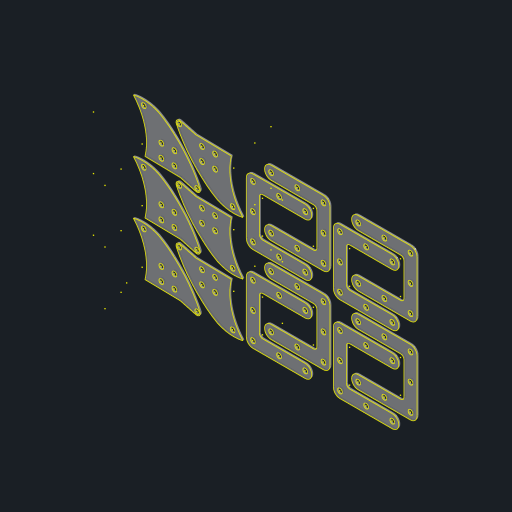
# Autodesk Inventor part: Nest.5-Sheet
Saved by Autodesk Inventor 2023 (Build 270158000, 158)
## iProperties
Created: 2023-05-16
Part Number: Nest.5-Sheet
Material: Polycarbonate, Clear
Document SubType Name: Modeling
Designer: reima
Density: 1.2 g/cm^3
Appearance: Polycarbonate - Clear
Author: reima
Autodesk Inventor part; units mm, degrees
ref_plane "YZ Plane" through (0, 0, 0) normal (1, 0, 0) x (0, 1, 0)
ref_plane "XZ Plane" through (0, 0, 0) normal (0, 1, 0) x (-1, 0, 0)
ref_plane "XY Plane" through (0, 0, 0) normal (0, 0, 1) x (1, 0, 0)
sketch "sleds sketch" plane through (0, 0, 0) normal (0, 0, 1) x (1, 0, 0)
  circle A0 centre (33.4038, 17.9574) radius 2.3114
  circle A1 centre (46.1038, 17.9574) radius 2.3114
  circle A2 centre (46.1038, 30.6574) radius 2.3114
  circle A3 centre (33.4038, 30.6574) radius 2.3114
  circle A4 centre (16.3571, 53.6521) radius 2.286
  circle A5 centre (68.0682, 9.9814) radius 2.159
  arc A6 (31.137, 55.194) -> (6.35, 57.7528) centre (15.0465, 20.661) ccw
  arc A7 (45.8139, 44.5419) -> (31.137, 55.194) centre (-5.4134, -10.6039) ccw
  arc A8 (70.9384, 11.3388) -> (45.8139, 44.5419) centre (-21.0694, -32.1754) ccw
  arc A9 (67.2386, 6.9167) -> (70.9384, 11.3388) centre (68.0682, 9.9814) ccw
  line L0 (67.2386, 6.9167) -> (51.9362, 11.059)
  line L1 (51.9362, 11.059) -> (17.5779, 11.7169)
  arc A10 (17.5779, 11.7169) -> (6.35, 57.7528) centre (-32.185, 23.9671) ccw
  constraints: 11 centre point, 10 point on circle, 4 end point
extrude "sleds extrude" add sketch "sleds sketch" along normal blind 1.5875
sketch "sleds (#2) sketch" plane through (0, 0, 0) normal (0, 0, 1) x (1, 0, 0)
  circle A0 centre (33.4038, 69.7529) radius 2.3114
  circle A1 centre (46.1038, 69.7529) radius 2.3114
  circle A2 centre (46.1038, 82.4529) radius 2.3114
  circle A3 centre (33.4038, 82.4529) radius 2.3114
  circle A4 centre (16.3571, 105.4475) radius 2.286
  circle A5 centre (68.0682, 61.7769) radius 2.159
  arc A6 (31.137, 106.9895) -> (6.35, 109.5483) centre (15.0465, 72.4565) ccw
  arc A7 (45.8139, 96.3374) -> (31.137, 106.9895) centre (-5.4134, 41.1916) ccw
  arc A8 (70.9384, 63.1343) -> (45.8139, 96.3374) centre (-21.0694, 19.6201) ccw
  arc A9 (67.2386, 58.7122) -> (70.9384, 63.1343) centre (68.0682, 61.7769) ccw
  line L0 (67.2386, 58.7122) -> (51.9362, 62.8545)
  line L1 (51.9362, 62.8545) -> (17.5779, 63.5124)
  arc A10 (17.5779, 63.5124) -> (6.35, 109.5483) centre (-32.185, 75.7626) ccw
  constraints: 11 centre point, 10 point on circle, 4 end point
extrude "sleds (#2) extrude" add sketch "sleds (#2) sketch" along normal blind 1.5875 separate body
sketch "sleds (#3) sketch" plane through (0, 0, 0) normal (0, 0, 1) x (1, 0, 0)
  circle A0 centre (33.4038, 121.5484) radius 2.3114
  circle A1 centre (46.1038, 121.5484) radius 2.3114
  circle A2 centre (46.1038, 134.2484) radius 2.3114
  circle A3 centre (33.4038, 134.2484) radius 2.3114
  circle A4 centre (16.3571, 157.243) radius 2.286
  circle A5 centre (68.0682, 113.5724) radius 2.159
  arc A6 (31.137, 158.785) -> (6.35, 161.3438) centre (15.0465, 124.252) ccw
  arc A7 (45.8139, 148.1329) -> (31.137, 158.785) centre (-5.4134, 92.9871) ccw
  arc A8 (70.9384, 114.9298) -> (45.8139, 148.1329) centre (-21.0694, 71.4156) ccw
  arc A9 (67.2386, 110.5077) -> (70.9384, 114.9298) centre (68.0682, 113.5724) ccw
  line L0 (67.2386, 110.5077) -> (51.9362, 114.6499)
  line L1 (51.9362, 114.6499) -> (17.5779, 115.3079)
  arc A10 (17.5779, 115.3079) -> (6.35, 161.3438) centre (-32.185, 127.5581) ccw
  constraints: 11 centre point, 10 point on circle, 4 end point
extrude "sleds (#3) extrude" add sketch "sleds (#3) sketch" along normal blind 1.5875 separate body
sketch "sleds (#4) sketch" plane through (0, 0, 0) normal (0, 0, 1) x (1, 0, 0)
  circle A0 centre (85.5586, 47.6077) radius 2.3114
  circle A1 centre (72.8586, 47.6077) radius 2.3114
  circle A2 centre (72.8586, 34.9077) radius 2.3114
  circle A3 centre (85.5586, 34.9077) radius 2.3114
  circle A4 centre (102.6053, 11.913) radius 2.286
  circle A5 centre (50.8942, 55.5837) radius 2.159
  arc A6 (87.8254, 10.3711) -> (112.6124, 7.8123) centre (103.9159, 44.9041) ccw
  arc A7 (73.1485, 21.0232) -> (87.8254, 10.3711) centre (124.3758, 76.169) ccw
  arc A8 (48.024, 54.2263) -> (73.1485, 21.0232) centre (140.0318, 97.7405) ccw
  arc A9 (51.7238, 58.6484) -> (48.024, 54.2263) centre (50.8942, 55.5837) ccw
  line L0 (51.7238, 58.6484) -> (67.0262, 54.5061)
  line L1 (67.0262, 54.5061) -> (101.3845, 53.8482)
  arc A10 (101.3845, 53.8482) -> (112.6124, 7.8123) centre (151.1474, 41.598) ccw
  constraints: 11 centre point, 10 point on circle, 4 end point
extrude "sleds (#4) extrude" add sketch "sleds (#4) sketch" along normal blind 1.5875 separate body
sketch "sleds (#5) sketch" plane through (0, 0, 0) normal (0, 0, 1) x (1, 0, 0)
  circle A0 centre (85.5586, 99.4032) radius 2.3114
  circle A1 centre (72.8586, 99.4032) radius 2.3114
  circle A2 centre (72.8586, 86.7032) radius 2.3114
  circle A3 centre (85.5586, 86.7032) radius 2.3114
  circle A4 centre (102.6053, 63.7085) radius 2.286
  circle A5 centre (50.8942, 107.3792) radius 2.159
  arc A6 (87.8254, 62.1666) -> (112.6124, 59.6077) centre (103.9159, 96.6996) ccw
  arc A7 (73.1485, 72.8187) -> (87.8254, 62.1666) centre (124.3758, 127.9645) ccw
  arc A8 (48.024, 106.0218) -> (73.1485, 72.8187) centre (140.0318, 149.536) ccw
  arc A9 (51.7238, 110.4439) -> (48.024, 106.0218) centre (50.8942, 107.3792) ccw
  line L0 (51.7238, 110.4439) -> (67.0262, 106.3016)
  line L1 (67.0262, 106.3016) -> (101.3845, 105.6437)
  arc A10 (101.3845, 105.6437) -> (112.6124, 59.6077) centre (151.1474, 93.3934) ccw
  constraints: 11 centre point, 10 point on circle, 4 end point
extrude "sleds (#5) extrude" add sketch "sleds (#5) sketch" along normal blind 1.5875 separate body
sketch "sleds (#6) sketch" plane through (0, 0, 0) normal (0, 0, 1) x (1, 0, 0)
  circle A0 centre (85.5586, 151.1987) radius 2.3114
  circle A1 centre (72.8586, 151.1987) radius 2.3114
  circle A2 centre (72.8586, 138.4987) radius 2.3114
  circle A3 centre (85.5586, 138.4987) radius 2.3114
  circle A4 centre (102.6053, 115.504) radius 2.286
  circle A5 centre (50.8942, 159.1747) radius 2.159
  arc A6 (87.8254, 113.9621) -> (112.6124, 111.4032) centre (103.9159, 148.4951) ccw
  arc A7 (73.1485, 124.6142) -> (87.8254, 113.9621) centre (124.3758, 179.76) ccw
  arc A8 (48.024, 157.8173) -> (73.1485, 124.6142) centre (140.0318, 201.3315) ccw
  arc A9 (51.7238, 162.2394) -> (48.024, 157.8173) centre (50.8942, 159.1747) ccw
  line L0 (51.7238, 162.2394) -> (67.0262, 158.0971)
  line L1 (67.0262, 158.0971) -> (101.3845, 157.4392)
  arc A10 (101.3845, 157.4392) -> (112.6124, 111.4032) centre (151.1474, 145.1889) ccw
  constraints: 11 centre point, 10 point on circle, 4 end point
extrude "sleds (#6) extrude" add sketch "sleds (#6) sketch" along normal blind 1.5875 separate body
sketch "frontgusset sketch" plane through (0, 0, 0) normal (0, 0, 1) x (1, 0, 0)
  circle A0 centre (147.6644, 63.5) radius 2.3368
  circle A1 centre (147.6644, 12.7) radius 2.3368
  circle A2 centre (122.2644, 38.1) radius 2.3368
  circle A3 centre (122.2644, 63.5) radius 2.3114
  circle A4 centre (173.0644, 63.5) radius 2.3114
  circle A5 centre (122.2644, 12.7) radius 2.3114
  circle A6 centre (173.0644, 12.7) radius 2.3114
  arc A7 (115.9144, 12.7) -> (122.2644, 6.35) centre (122.2644, 12.7) ccw
  line L0 (115.9144, 12.7) -> (115.9144, 63.5)
  arc A8 (122.2644, 69.85) -> (115.9144, 63.5) centre (122.2644, 63.5) ccw
  line L1 (122.2644, 69.85) -> (173.0644, 69.85)
  arc A9 (173.0644, 57.15) -> (173.0644, 69.85) centre (173.0644, 63.5) ccw
  line L2 (173.0644, 57.15) -> (131.7894, 57.15)
  arc A10 (131.7894, 57.15) -> (128.6144, 53.975) centre (131.7894, 53.975) ccw
  line L3 (128.6144, 53.975) -> (128.6144, 22.225)
  arc A11 (128.6144, 22.225) -> (131.7894, 19.05) centre (131.7894, 22.225) ccw
  line L4 (131.7894, 19.05) -> (173.0644, 19.05)
  arc A12 (173.0644, 6.35) -> (173.0644, 19.05) centre (173.0644, 12.7) ccw
  line L5 (173.0644, 6.35) -> (122.2644, 6.35)
  constraints: 13 centre point, 12 end point, 12 point on circle
extrude "frontgusset extrude" add sketch "frontgusset sketch" along normal blind 1.5875 separate body
sketch "frontgusset (#2) sketch" plane through (0, 0, 0) normal (0, 0, 1) x (1, 0, 0)
  circle A0 centre (165.3571, 28.9148) radius 2.3368
  circle A1 centre (165.3571, 79.7148) radius 2.3368
  circle A2 centre (190.7571, 54.3148) radius 2.3368
  circle A3 centre (190.7571, 28.9148) radius 2.3114
  circle A4 centre (139.9571, 28.9148) radius 2.3114
  circle A5 centre (190.7571, 79.7148) radius 2.3114
  circle A6 centre (139.9571, 79.7148) radius 2.3114
  arc A7 (197.1071, 79.7148) -> (190.7571, 86.0648) centre (190.7571, 79.7148) ccw
  line L0 (197.1071, 79.7148) -> (197.1071, 28.9148)
  arc A8 (190.7571, 22.5648) -> (197.1071, 28.9148) centre (190.7571, 28.9149) ccw
  line L1 (190.7571, 22.5648) -> (139.9571, 22.5648)
  arc A9 (139.9571, 35.2649) -> (139.9571, 22.5648) centre (139.9571, 28.9149) ccw
  line L2 (139.9571, 35.2649) -> (181.2321, 35.2649)
  arc A10 (181.2321, 35.2649) -> (184.4071, 38.4398) centre (181.2321, 38.4398) ccw
  line L3 (184.4071, 38.4398) -> (184.4071, 70.1898)
  arc A11 (184.4071, 70.1898) -> (181.2321, 73.3649) centre (181.2321, 70.1899) ccw
  line L4 (181.2321, 73.3649) -> (139.9571, 73.3649)
  arc A12 (139.9571, 86.0648) -> (139.9571, 73.3649) centre (139.9571, 79.7149) ccw
  line L5 (139.9571, 86.0648) -> (190.7571, 86.0648)
  constraints: 13 centre point, 12 end point, 12 point on circle
extrude "frontgusset (#2) extrude" add sketch "frontgusset (#2) sketch" along normal blind 1.5875 separate body
sketch "frontgusset (#3) sketch" plane through (0, 0, 0) normal (0, 0, 1) x (1, 0, 0)
  circle A0 centre (147.6644, 146.5169) radius 2.3368
  circle A1 centre (147.6644, 95.7169) radius 2.3368
  circle A2 centre (122.2644, 121.1169) radius 2.3368
  circle A3 centre (122.2644, 146.5168) radius 2.3114
  circle A4 centre (173.0644, 146.5169) radius 2.3114
  circle A5 centre (122.2644, 95.7169) radius 2.3114
  circle A6 centre (173.0644, 95.7169) radius 2.3114
  arc A7 (115.9144, 95.7169) -> (122.2644, 89.3669) centre (122.2644, 95.7169) ccw
  line L0 (115.9144, 95.7169) -> (115.9144, 146.5168)
  arc A8 (122.2644, 152.8669) -> (115.9144, 146.5168) centre (122.2644, 146.5168) ccw
  line L1 (122.2644, 152.8669) -> (173.0644, 152.8669)
  arc A9 (173.0644, 140.1669) -> (173.0644, 152.8669) centre (173.0644, 146.5169) ccw
  line L2 (173.0644, 140.1669) -> (131.7894, 140.1668)
  arc A10 (131.7894, 140.1668) -> (128.6144, 136.9919) centre (131.7894, 136.9918) ccw
  line L3 (128.6144, 136.9919) -> (128.6144, 105.2419)
  arc A11 (128.6144, 105.2419) -> (131.7894, 102.0669) centre (131.7894, 105.2419) ccw
  line L4 (131.7894, 102.0669) -> (173.0644, 102.0669)
  arc A12 (173.0644, 89.3669) -> (173.0644, 102.0669) centre (173.0644, 95.7169) ccw
  line L5 (173.0644, 89.3669) -> (122.2644, 89.3669)
  constraints: 13 centre point, 12 end point, 12 point on circle
extrude "frontgusset (#3) extrude" add sketch "frontgusset (#3) sketch" along normal blind 1.5875 separate body
sketch "frontgusset (#4) sketch" plane through (0, 0, 0) normal (0, 0, 1) x (1, 0, 0)
  circle A0 centre (165.3571, 111.9317) radius 2.3368
  circle A1 centre (165.3571, 162.7317) radius 2.3368
  circle A2 centre (190.7571, 137.3317) radius 2.3368
  circle A3 centre (190.7571, 111.9317) radius 2.3114
  circle A4 centre (139.9571, 111.9317) radius 2.3114
  circle A5 centre (190.7571, 162.7317) radius 2.3114
  circle A6 centre (139.9571, 162.7317) radius 2.3114
  arc A7 (197.1071, 162.7317) -> (190.7571, 169.0817) centre (190.7571, 162.7317) ccw
  line L0 (197.1071, 162.7317) -> (197.1071, 111.9317)
  arc A8 (190.7571, 105.5817) -> (197.1071, 111.9317) centre (190.7571, 111.9317) ccw
  line L1 (190.7571, 105.5817) -> (139.9571, 105.5817)
  arc A9 (139.9571, 118.2817) -> (139.9571, 105.5817) centre (139.9571, 111.9317) ccw
  line L2 (139.9571, 118.2817) -> (181.2321, 118.2817)
  arc A10 (181.2321, 118.2817) -> (184.4071, 121.4567) centre (181.2321, 121.4567) ccw
  line L3 (184.4071, 121.4567) -> (184.4071, 153.2067)
  arc A11 (184.4071, 153.2067) -> (181.2321, 156.3817) centre (181.2321, 153.2067) ccw
  line L4 (181.2321, 156.3817) -> (139.9571, 156.3817)
  arc A12 (139.9571, 169.0817) -> (139.9571, 156.3817) centre (139.9571, 162.7317) ccw
  line L5 (139.9571, 169.0817) -> (190.7571, 169.0817)
  constraints: 13 centre point, 12 end point, 12 point on circle
extrude "frontgusset (#4) extrude" add sketch "frontgusset (#4) sketch" along normal blind 1.5875 separate body
sketch "frontgusset (#5) sketch" plane through (0, 0, 0) normal (0, 0, 1) x (1, 0, 0)
  circle A0 centre (232.1591, 63.5) radius 2.3368
  circle A1 centre (232.1591, 12.7) radius 2.3368
  circle A2 centre (206.7591, 38.1) radius 2.3368
  circle A3 centre (206.7591, 63.5) radius 2.3114
  circle A4 centre (257.5591, 63.5) radius 2.3114
  circle A5 centre (206.7591, 12.7) radius 2.3114
  circle A6 centre (257.5591, 12.7) radius 2.3114
  arc A7 (200.4091, 12.7) -> (206.7591, 6.35) centre (206.7591, 12.7) ccw
  line L0 (200.4091, 12.7) -> (200.4091, 63.5)
  arc A8 (206.7591, 69.85) -> (200.4091, 63.5) centre (206.7591, 63.5) ccw
  line L1 (206.7591, 69.85) -> (257.5591, 69.85)
  arc A9 (257.5591, 57.15) -> (257.5591, 69.85) centre (257.5591, 63.5) ccw
  line L2 (257.5591, 57.15) -> (216.2841, 57.15)
  arc A10 (216.2841, 57.15) -> (213.1091, 53.975) centre (216.2841, 53.975) ccw
  line L3 (213.1091, 53.975) -> (213.1091, 22.225)
  arc A11 (213.1091, 22.225) -> (216.2841, 19.05) centre (216.2841, 22.225) ccw
  line L4 (216.2841, 19.05) -> (257.5591, 19.05)
  arc A12 (257.5591, 6.35) -> (257.5591, 19.05) centre (257.5591, 12.7) ccw
  line L5 (257.5591, 6.35) -> (206.7591, 6.35)
  constraints: 13 centre point, 12 end point, 12 point on circle
extrude "frontgusset (#5) extrude" add sketch "frontgusset (#5) sketch" along normal blind 1.5875 separate body
sketch "frontgusset (#6) sketch" plane through (0, 0, 0) normal (0, 0, 1) x (1, 0, 0)
  circle A0 centre (249.8518, 28.9148) radius 2.3368
  circle A1 centre (249.8518, 79.7148) radius 2.3368
  circle A2 centre (275.2518, 54.3148) radius 2.3368
  circle A3 centre (275.2518, 28.9148) radius 2.3114
  circle A4 centre (224.4518, 28.9148) radius 2.3114
  circle A5 centre (275.2518, 79.7148) radius 2.3114
  circle A6 centre (224.4518, 79.7148) radius 2.3114
  arc A7 (281.6018, 79.7148) -> (275.2518, 86.0648) centre (275.2518, 79.7148) ccw
  line L0 (281.6018, 79.7148) -> (281.6018, 28.9148)
  arc A8 (275.2518, 22.5648) -> (281.6018, 28.9148) centre (275.2518, 28.9149) ccw
  line L1 (275.2518, 22.5648) -> (224.4518, 22.5648)
  arc A9 (224.4518, 35.2649) -> (224.4518, 22.5648) centre (224.4518, 28.9149) ccw
  line L2 (224.4518, 35.2649) -> (265.7268, 35.2649)
  arc A10 (265.7268, 35.2649) -> (268.9018, 38.4398) centre (265.7268, 38.4398) ccw
  line L3 (268.9018, 38.4398) -> (268.9018, 70.1898)
  arc A11 (268.9018, 70.1898) -> (265.7268, 73.3649) centre (265.7268, 70.1899) ccw
  line L4 (265.7268, 73.3649) -> (224.4518, 73.3649)
  arc A12 (224.4518, 86.0648) -> (224.4518, 73.3649) centre (224.4518, 79.7149) ccw
  line L5 (224.4518, 86.0648) -> (275.2518, 86.0648)
  constraints: 13 centre point, 12 end point, 12 point on circle
extrude "frontgusset (#6) extrude" add sketch "frontgusset (#6) sketch" along normal blind 1.5875 separate body
sketch "frontgusset (#7) sketch" plane through (0, 0, 0) normal (0, 0, 1) x (1, 0, 0)
  circle A0 centre (232.1591, 146.5169) radius 2.3368
  circle A1 centre (232.1591, 95.7169) radius 2.3368
  circle A2 centre (206.7591, 121.1169) radius 2.3368
  circle A3 centre (206.7591, 146.5168) radius 2.3114
  circle A4 centre (257.5591, 146.5169) radius 2.3114
  circle A5 centre (206.7591, 95.7169) radius 2.3114
  circle A6 centre (257.5591, 95.7169) radius 2.3114
  arc A7 (200.4091, 95.7169) -> (206.7591, 89.3669) centre (206.7591, 95.7169) ccw
  line L0 (200.4091, 95.7169) -> (200.4091, 146.5168)
  arc A8 (206.7591, 152.8669) -> (200.4091, 146.5168) centre (206.7591, 146.5168) ccw
  line L1 (206.7591, 152.8669) -> (257.5591, 152.8669)
  arc A9 (257.5591, 140.1669) -> (257.5591, 152.8669) centre (257.5591, 146.5169) ccw
  line L2 (257.5591, 140.1669) -> (216.2841, 140.1668)
  arc A10 (216.2841, 140.1668) -> (213.1091, 136.9919) centre (216.2841, 136.9918) ccw
  line L3 (213.1091, 136.9919) -> (213.1091, 105.2419)
  arc A11 (213.1091, 105.2419) -> (216.2841, 102.0669) centre (216.2841, 105.2419) ccw
  line L4 (216.2841, 102.0669) -> (257.5591, 102.0669)
  arc A12 (257.5591, 89.3669) -> (257.5591, 102.0669) centre (257.5591, 95.7169) ccw
  line L5 (257.5591, 89.3669) -> (206.7591, 89.3669)
  constraints: 13 centre point, 12 end point, 12 point on circle
extrude "frontgusset (#7) extrude" add sketch "frontgusset (#7) sketch" along normal blind 1.5875 separate body
sketch "frontgusset (#8) sketch" plane through (0, 0, 0) normal (0, 0, 1) x (1, 0, 0)
  circle A0 centre (249.8518, 111.9317) radius 2.3368
  circle A1 centre (249.8518, 162.7317) radius 2.3368
  circle A2 centre (275.2518, 137.3317) radius 2.3368
  circle A3 centre (275.2518, 111.9317) radius 2.3114
  circle A4 centre (224.4518, 111.9317) radius 2.3114
  circle A5 centre (275.2518, 162.7317) radius 2.3114
  circle A6 centre (224.4518, 162.7317) radius 2.3114
  arc A7 (281.6018, 162.7317) -> (275.2518, 169.0817) centre (275.2518, 162.7317) ccw
  line L0 (281.6018, 162.7317) -> (281.6018, 111.9317)
  arc A8 (275.2518, 105.5817) -> (281.6018, 111.9317) centre (275.2518, 111.9317) ccw
  line L1 (275.2518, 105.5817) -> (224.4518, 105.5817)
  arc A9 (224.4518, 118.2817) -> (224.4518, 105.5817) centre (224.4518, 111.9317) ccw
  line L2 (224.4518, 118.2817) -> (265.7268, 118.2817)
  arc A10 (265.7268, 118.2817) -> (268.9018, 121.4567) centre (265.7268, 121.4567) ccw
  line L3 (268.9018, 121.4567) -> (268.9018, 153.2067)
  arc A11 (268.9018, 153.2067) -> (265.7268, 156.3817) centre (265.7268, 153.2067) ccw
  line L4 (265.7268, 156.3817) -> (224.4518, 156.3817)
  arc A12 (224.4518, 169.0817) -> (224.4518, 156.3817) centre (224.4518, 162.7317) ccw
  line L5 (224.4518, 169.0817) -> (275.2518, 169.0817)
  constraints: 13 centre point, 12 end point, 12 point on circle
extrude "frontgusset (#8) extrude" add sketch "frontgusset (#8) sketch" along normal blind 1.5875 separate body
sketch "Sketch16" plane through (0, 0, 1.5875) normal (0, 0, 1) x (1, 0, 0)
  circle A0 centre (33.4038, 134.2484) radius 2.3114 projected
  circle A1 centre (46.1038, 134.2484) radius 2.3114 projected
  circle A2 centre (46.1038, 121.5484) radius 2.3114 projected
  circle A3 centre (33.4038, 121.5484) radius 2.3114 projected
  circle A4 centre (16.3571, 157.243) radius 2.286 projected
  circle A5 centre (68.0682, 113.5724) radius 2.159 projected
  arc A6 (31.137, 158.785) -> (6.35, 161.3438) centre (15.0465, 124.252) ccw projected
  arc A7 (17.5779, 115.3079) -> (6.35, 161.3438) centre (-32.185, 127.5581) ccw projected
  line L0 (17.5779, 115.3079) -> (51.9362, 114.6499) projected
  line L1 (51.9362, 114.6499) -> (67.2386, 110.5077) projected
  arc A8 (67.2386, 110.5077) -> (70.9384, 114.9298) centre (68.0682, 113.5724) ccw projected
  arc A9 (70.9384, 114.9298) -> (45.8139, 148.1329) centre (-21.0694, 71.4156) ccw projected
  arc A10 (45.8139, 148.1329) -> (31.137, 158.785) centre (-5.4134, 92.9871) ccw projected
  circle A11 centre (85.5586, 138.4987) radius 2.3114 projected
  circle A12 centre (72.8586, 138.4987) radius 2.3114 projected
  circle A13 centre (72.8586, 151.1987) radius 2.3114 projected
  circle A14 centre (85.5586, 151.1987) radius 2.3114 projected
  circle A15 centre (102.6053, 115.504) radius 2.286 projected
  circle A16 centre (50.8942, 159.1747) radius 2.159 projected
  arc A17 (87.8254, 113.9621) -> (112.6124, 111.4032) centre (103.9159, 148.4951) ccw projected
  arc A18 (101.3845, 157.4392) -> (112.6124, 111.4032) centre (151.1474, 145.1889) ccw projected
  line L2 (101.3845, 157.4392) -> (67.0262, 158.0971) projected
  line L3 (67.0262, 158.0971) -> (51.7238, 162.2394) projected
  arc A19 (51.7238, 162.2394) -> (48.024, 157.8173) centre (50.8942, 159.1747) ccw projected
  arc A20 (48.024, 157.8173) -> (73.1485, 124.6142) centre (140.0318, 201.3315) ccw projected
  arc A21 (73.1485, 124.6142) -> (87.8254, 113.9621) centre (124.3758, 179.76) ccw projected
  circle A22 centre (122.2644, 121.1169) radius 2.3368 projected
  circle A23 centre (147.6644, 95.7169) radius 2.3368 projected
  circle A24 centre (147.6644, 146.5169) radius 2.3368 projected
  circle A25 centre (173.0644, 95.7169) radius 2.3114 projected
  circle A26 centre (122.2644, 95.7169) radius 2.3114 projected
  circle A27 centre (173.0644, 146.5169) radius 2.3114 projected
  circle A28 centre (122.2644, 146.5168) radius 2.3114 projected
  arc A29 (115.9144, 95.7169) -> (122.2644, 89.3669) centre (122.2644, 95.7169) ccw projected
  line L4 (122.2644, 89.3669) -> (173.0644, 89.3669) projected
  arc A30 (173.0644, 89.3669) -> (173.0644, 102.0669) centre (173.0644, 95.7169) ccw projected
  line L5 (173.0644, 102.0669) -> (131.7894, 102.0669) projected
  arc A31 (128.6144, 105.2419) -> (131.7894, 102.0669) centre (131.7894, 105.2419) ccw projected
  line L6 (128.6144, 105.2419) -> (128.6144, 136.9919) projected
  arc A32 (131.7894, 140.1668) -> (128.6144, 136.9919) centre (131.7894, 136.9918) ccw projected
  line L7 (131.7894, 140.1668) -> (173.0644, 140.1669) projected
  arc A33 (173.0644, 140.1669) -> (173.0644, 152.8669) centre (173.0644, 146.5169) ccw projected
  line L8 (173.0644, 152.8669) -> (122.2644, 152.8669) projected
  arc A34 (122.2644, 152.8669) -> (115.9144, 146.5168) centre (122.2644, 146.5168) ccw projected
  line L9 (115.9144, 146.5168) -> (115.9144, 95.7169) projected
  circle A35 centre (190.7571, 137.3317) radius 2.3368 projected
  circle A36 centre (165.3571, 162.7317) radius 2.3368 projected
  circle A37 centre (165.3571, 111.9317) radius 2.3368 projected
  circle A38 centre (139.9571, 162.7317) radius 2.3114 projected
  circle A39 centre (190.7571, 162.7317) radius 2.3114 projected
  circle A40 centre (139.9571, 111.9317) radius 2.3114 projected
  circle A41 centre (190.7571, 111.9317) radius 2.3114 projected
  arc A42 (197.1071, 162.7317) -> (190.7571, 169.0817) centre (190.7571, 162.7317) ccw projected
  line L10 (190.7571, 169.0817) -> (139.9571, 169.0817) projected
  arc A43 (139.9571, 169.0817) -> (139.9571, 156.3817) centre (139.9571, 162.7317) ccw projected
  line L11 (139.9571, 156.3817) -> (181.2321, 156.3817) projected
  arc A44 (184.4071, 153.2067) -> (181.2321, 156.3817) centre (181.2321, 153.2067) ccw projected
  line L12 (184.4071, 153.2067) -> (184.4071, 121.4567) projected
  arc A45 (181.2321, 118.2817) -> (184.4071, 121.4567) centre (181.2321, 121.4567) ccw projected
  line L13 (181.2321, 118.2817) -> (139.9571, 118.2817) projected
  arc A46 (139.9571, 118.2817) -> (139.9571, 105.5817) centre (139.9571, 111.9317) ccw projected
  line L14 (139.9571, 105.5817) -> (190.7571, 105.5817) projected
  arc A47 (190.7571, 105.5817) -> (197.1071, 111.9317) centre (190.7571, 111.9317) ccw projected
  line L15 (197.1071, 111.9317) -> (197.1071, 162.7317) projected
  circle A48 centre (206.7591, 121.1169) radius 2.3368 projected
  circle A49 centre (232.1591, 95.7169) radius 2.3368 projected
  circle A50 centre (232.1591, 146.5169) radius 2.3368 projected
  circle A51 centre (257.5591, 95.7169) radius 2.3114 projected
  circle A52 centre (206.7591, 95.7169) radius 2.3114 projected
  circle A53 centre (257.5591, 146.5169) radius 2.3114 projected
  circle A54 centre (206.7591, 146.5168) radius 2.3114 projected
  arc A55 (200.4091, 95.7169) -> (206.7591, 89.3669) centre (206.7591, 95.7169) ccw projected
  line L16 (206.7591, 89.3669) -> (257.5591, 89.3669) projected
  arc A56 (257.5591, 89.3669) -> (257.5591, 102.0669) centre (257.5591, 95.7169) ccw projected
  line L17 (257.5591, 102.0669) -> (216.2841, 102.0669) projected
  arc A57 (213.1091, 105.2419) -> (216.2841, 102.0669) centre (216.2841, 105.2419) ccw projected
  line L18 (213.1091, 105.2419) -> (213.1091, 136.9919) projected
  arc A58 (216.2841, 140.1668) -> (213.1091, 136.9919) centre (216.2841, 136.9918) ccw projected
  line L19 (216.2841, 140.1668) -> (257.5591, 140.1669) projected
  arc A59 (257.5591, 140.1669) -> (257.5591, 152.8669) centre (257.5591, 146.5169) ccw projected
  line L20 (257.5591, 152.8669) -> (206.7591, 152.8669) projected
  arc A60 (206.7591, 152.8669) -> (200.4091, 146.5168) centre (206.7591, 146.5168) ccw projected
  line L21 (200.4091, 146.5168) -> (200.4091, 95.7169) projected
  circle A61 centre (275.2518, 137.3317) radius 2.3368 projected
  circle A62 centre (249.8518, 162.7317) radius 2.3368 projected
  circle A63 centre (249.8518, 111.9317) radius 2.3368 projected
  circle A64 centre (224.4518, 162.7317) radius 2.3114 projected
  circle A65 centre (275.2518, 162.7317) radius 2.3114 projected
  circle A66 centre (224.4518, 111.9317) radius 2.3114 projected
  circle A67 centre (275.2518, 111.9317) radius 2.3114 projected
  arc A68 (281.6018, 162.7317) -> (275.2518, 169.0817) centre (275.2518, 162.7317) ccw projected
  line L22 (275.2518, 169.0817) -> (224.4518, 169.0817) projected
  arc A69 (224.4518, 169.0817) -> (224.4518, 156.3817) centre (224.4518, 162.7317) ccw projected
  line L23 (224.4518, 156.3817) -> (265.7268, 156.3817) projected
  arc A70 (268.9018, 153.2067) -> (265.7268, 156.3817) centre (265.7268, 153.2067) ccw projected
  line L24 (268.9018, 153.2067) -> (268.9018, 121.4567) projected
  arc A71 (265.7268, 118.2817) -> (268.9018, 121.4567) centre (265.7268, 121.4567) ccw projected
  line L25 (265.7268, 118.2817) -> (224.4518, 118.2817) projected
  arc A72 (224.4518, 118.2817) -> (224.4518, 105.5817) centre (224.4518, 111.9317) ccw projected
  line L26 (224.4518, 105.5817) -> (275.2518, 105.5817) projected
  arc A73 (275.2518, 105.5817) -> (281.6018, 111.9317) centre (275.2518, 111.9317) ccw projected
  line L27 (281.6018, 111.9317) -> (281.6018, 162.7317) projected
  circle A74 centre (275.2518, 54.3148) radius 2.3368 projected
  circle A75 centre (249.8518, 79.7148) radius 2.3368 projected
  circle A76 centre (249.8518, 28.9148) radius 2.3368 projected
  circle A77 centre (224.4518, 79.7148) radius 2.3114 projected
  circle A78 centre (275.2518, 79.7148) radius 2.3114 projected
  circle A79 centre (224.4518, 28.9148) radius 2.3114 projected
  circle A80 centre (275.2518, 28.9148) radius 2.3114 projected
  arc A81 (281.6018, 79.7148) -> (275.2518, 86.0648) centre (275.2518, 79.7148) ccw projected
  line L28 (275.2518, 86.0648) -> (224.4518, 86.0648) projected
  arc A82 (224.4518, 86.0648) -> (224.4518, 73.3649) centre (224.4518, 79.7149) ccw projected
  line L29 (224.4518, 73.3649) -> (265.7268, 73.3649) projected
  arc A83 (268.9018, 70.1898) -> (265.7268, 73.3649) centre (265.7268, 70.1899) ccw projected
  line L30 (268.9018, 70.1898) -> (268.9018, 38.4398) projected
  arc A84 (265.7268, 35.2649) -> (268.9018, 38.4398) centre (265.7268, 38.4398) ccw projected
  line L31 (265.7268, 35.2649) -> (224.4518, 35.2649) projected
  arc A85 (224.4518, 35.2649) -> (224.4518, 22.5648) centre (224.4518, 28.9149) ccw projected
  line L32 (224.4518, 22.5648) -> (275.2518, 22.5648) projected
  arc A86 (275.2518, 22.5648) -> (281.6018, 28.9148) centre (275.2518, 28.9149) ccw projected
  line L33 (281.6018, 28.9148) -> (281.6018, 79.7148) projected
  circle A87 centre (206.7591, 38.1) radius 2.3368 projected
  circle A88 centre (232.1591, 12.7) radius 2.3368 projected
  circle A89 centre (232.1591, 63.5) radius 2.3368 projected
  circle A90 centre (257.5591, 12.7) radius 2.3114 projected
  circle A91 centre (206.7591, 12.7) radius 2.3114 projected
  circle A92 centre (257.5591, 63.5) radius 2.3114 projected
  circle A93 centre (206.7591, 63.5) radius 2.3114 projected
  arc A94 (200.4091, 12.7) -> (206.7591, 6.35) centre (206.7591, 12.7) ccw projected
  line L34 (206.7591, 6.35) -> (257.5591, 6.35) projected
  arc A95 (257.5591, 6.35) -> (257.5591, 19.05) centre (257.5591, 12.7) ccw projected
  line L35 (257.5591, 19.05) -> (216.2841, 19.05) projected
  arc A96 (213.1091, 22.225) -> (216.2841, 19.05) centre (216.2841, 22.225) ccw projected
  line L36 (213.1091, 22.225) -> (213.1091, 53.975) projected
  arc A97 (216.2841, 57.15) -> (213.1091, 53.975) centre (216.2841, 53.975) ccw projected
  line L37 (216.2841, 57.15) -> (257.5591, 57.15) projected
  arc A98 (257.5591, 57.15) -> (257.5591, 69.85) centre (257.5591, 63.5) ccw projected
  line L38 (257.5591, 69.85) -> (206.7591, 69.85) projected
  arc A99 (206.7591, 69.85) -> (200.4091, 63.5) centre (206.7591, 63.5) ccw projected
  line L39 (200.4091, 63.5) -> (200.4091, 12.7) projected
  circle A100 centre (190.7571, 54.3148) radius 2.3368 projected
  circle A101 centre (165.3571, 79.7148) radius 2.3368 projected
  circle A102 centre (165.3571, 28.9148) radius 2.3368 projected
  circle A103 centre (139.9571, 79.7148) radius 2.3114 projected
  circle A104 centre (190.7571, 79.7148) radius 2.3114 projected
  circle A105 centre (139.9571, 28.9148) radius 2.3114 projected
  circle A106 centre (190.7571, 28.9148) radius 2.3114 projected
  arc A107 (197.1071, 79.7148) -> (190.7571, 86.0648) centre (190.7571, 79.7148) ccw projected
  line L40 (190.7571, 86.0648) -> (139.9571, 86.0648) projected
  arc A108 (139.9571, 86.0648) -> (139.9571, 73.3649) centre (139.9571, 79.7149) ccw projected
  line L41 (139.9571, 73.3649) -> (181.2321, 73.3649) projected
  arc A109 (184.4071, 70.1898) -> (181.2321, 73.3649) centre (181.2321, 70.1899) ccw projected
  line L42 (184.4071, 70.1898) -> (184.4071, 38.4398) projected
  arc A110 (181.2321, 35.2649) -> (184.4071, 38.4398) centre (181.2321, 38.4398) ccw projected
  line L43 (181.2321, 35.2649) -> (139.9571, 35.2649) projected
  arc A111 (139.9571, 35.2649) -> (139.9571, 22.5648) centre (139.9571, 28.9149) ccw projected
  line L44 (139.9571, 22.5648) -> (190.7571, 22.5648) projected
  arc A112 (190.7571, 22.5648) -> (197.1071, 28.9148) centre (190.7571, 28.9149) ccw projected
  line L45 (197.1071, 28.9148) -> (197.1071, 79.7148) projected
  circle A113 centre (122.2644, 38.1) radius 2.3368 projected
  circle A114 centre (147.6644, 12.7) radius 2.3368 projected
  circle A115 centre (147.6644, 63.5) radius 2.3368 projected
  circle A116 centre (173.0644, 12.7) radius 2.3114 projected
  circle A117 centre (122.2644, 12.7) radius 2.3114 projected
  circle A118 centre (173.0644, 63.5) radius 2.3114 projected
  circle A119 centre (122.2644, 63.5) radius 2.3114 projected
  arc A120 (115.9144, 12.7) -> (122.2644, 6.35) centre (122.2644, 12.7) ccw projected
  line L46 (122.2644, 6.35) -> (173.0644, 6.35) projected
  arc A121 (173.0644, 6.35) -> (173.0644, 19.05) centre (173.0644, 12.7) ccw projected
  line L47 (173.0644, 19.05) -> (131.7894, 19.05) projected
  arc A122 (128.6144, 22.225) -> (131.7894, 19.05) centre (131.7894, 22.225) ccw projected
  line L48 (128.6144, 22.225) -> (128.6144, 53.975) projected
  arc A123 (131.7894, 57.15) -> (128.6144, 53.975) centre (131.7894, 53.975) ccw projected
  line L49 (131.7894, 57.15) -> (173.0644, 57.15) projected
  arc A124 (173.0644, 57.15) -> (173.0644, 69.85) centre (173.0644, 63.5) ccw projected
  line L50 (173.0644, 69.85) -> (122.2644, 69.85) projected
  arc A125 (122.2644, 69.85) -> (115.9144, 63.5) centre (122.2644, 63.5) ccw projected
  line L51 (115.9144, 63.5) -> (115.9144, 12.7) projected
  circle A126 centre (85.5586, 34.9077) radius 2.3114 projected
  circle A127 centre (72.8586, 34.9077) radius 2.3114 projected
  circle A128 centre (72.8586, 47.6077) radius 2.3114 projected
  circle A129 centre (85.5586, 47.6077) radius 2.3114 projected
  circle A130 centre (102.6053, 11.913) radius 2.286 projected
  circle A131 centre (50.8942, 55.5837) radius 2.159 projected
  arc A132 (87.8254, 10.3711) -> (112.6124, 7.8123) centre (103.9159, 44.9041) ccw projected
  arc A133 (101.3845, 53.8482) -> (112.6124, 7.8123) centre (151.1474, 41.598) ccw projected
  line L52 (101.3845, 53.8482) -> (67.0262, 54.5061) projected
  line L53 (67.0262, 54.5061) -> (51.7238, 58.6484) projected
  arc A134 (51.7238, 58.6484) -> (48.024, 54.2263) centre (50.8942, 55.5837) ccw projected
  arc A135 (48.024, 54.2263) -> (73.1485, 21.0232) centre (140.0318, 97.7405) ccw projected
  arc A136 (73.1485, 21.0232) -> (87.8254, 10.3711) centre (124.3758, 76.169) ccw projected
  circle A137 centre (85.5586, 86.7032) radius 2.3114 projected
  circle A138 centre (72.8586, 86.7032) radius 2.3114 projected
  circle A139 centre (72.8586, 99.4032) radius 2.3114 projected
  circle A140 centre (85.5586, 99.4032) radius 2.3114 projected
  circle A141 centre (102.6053, 63.7085) radius 2.286 projected
  circle A142 centre (50.8942, 107.3792) radius 2.159 projected
  arc A143 (87.8254, 62.1666) -> (112.6124, 59.6077) centre (103.9159, 96.6996) ccw projected
  arc A144 (101.3845, 105.6437) -> (112.6124, 59.6077) centre (151.1474, 93.3934) ccw projected
  line L54 (101.3845, 105.6437) -> (67.0262, 106.3016) projected
  line L55 (67.0262, 106.3016) -> (51.7238, 110.4439) projected
  arc A145 (51.7238, 110.4439) -> (48.024, 106.0218) centre (50.8942, 107.3792) ccw projected
  arc A146 (48.024, 106.0218) -> (73.1485, 72.8187) centre (140.0318, 149.536) ccw projected
  arc A147 (73.1485, 72.8187) -> (87.8254, 62.1666) centre (124.3758, 127.9645) ccw projected
  circle A148 centre (33.4038, 82.4529) radius 2.3114 projected
  circle A149 centre (46.1038, 82.4529) radius 2.3114 projected
  circle A150 centre (46.1038, 69.7529) radius 2.3114 projected
  circle A151 centre (33.4038, 69.7529) radius 2.3114 projected
  circle A152 centre (16.3571, 105.4475) radius 2.286 projected
  circle A153 centre (68.0682, 61.7769) radius 2.159 projected
  arc A154 (31.137, 106.9895) -> (6.35, 109.5483) centre (15.0465, 72.4565) ccw projected
  arc A155 (17.5779, 63.5124) -> (6.35, 109.5483) centre (-32.185, 75.7626) ccw projected
  line L56 (17.5779, 63.5124) -> (51.9362, 62.8545) projected
  line L57 (51.9362, 62.8545) -> (67.2386, 58.7122) projected
  arc A156 (67.2386, 58.7122) -> (70.9384, 63.1343) centre (68.0682, 61.7769) ccw projected
  arc A157 (70.9384, 63.1343) -> (45.8139, 96.3374) centre (-21.0694, 19.6201) ccw projected
  arc A158 (45.8139, 96.3374) -> (31.137, 106.9895) centre (-5.4134, 41.1916) ccw projected
  circle A159 centre (33.4038, 30.6574) radius 2.3114 projected
  circle A160 centre (46.1038, 30.6574) radius 2.3114 projected
  circle A161 centre (46.1038, 17.9574) radius 2.3114 projected
  circle A162 centre (33.4038, 17.9574) radius 2.3114 projected
  circle A163 centre (16.3571, 53.6521) radius 2.286 projected
  circle A164 centre (68.0682, 9.9814) radius 2.159 projected
  arc A165 (31.137, 55.194) -> (6.35, 57.7528) centre (15.0465, 20.661) ccw projected
  arc A166 (17.5779, 11.7169) -> (6.35, 57.7528) centre (-32.185, 23.9671) ccw projected
  line L58 (17.5779, 11.7169) -> (51.9362, 11.059) projected
  line L59 (51.9362, 11.059) -> (67.2386, 6.9167) projected
  arc A167 (67.2386, 6.9167) -> (70.9384, 11.3388) centre (68.0682, 9.9814) ccw projected
  arc A168 (70.9384, 11.3388) -> (45.8139, 44.5419) centre (-21.0694, -32.1754) ccw projected
  arc A169 (45.8139, 44.5419) -> (31.137, 55.194) centre (-5.4134, -10.6039) ccw projected
  point P0 (0, 0)
